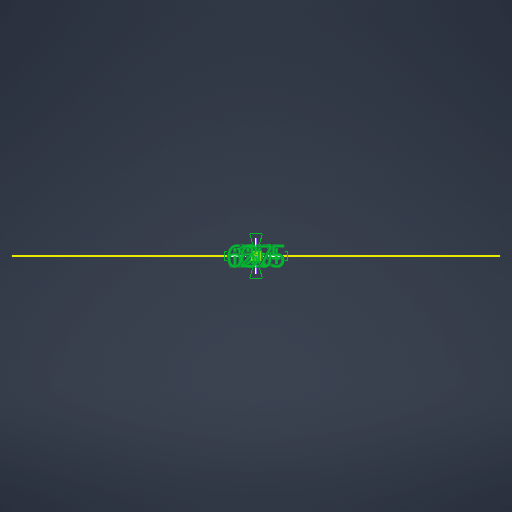
# Autodesk Inventor part: Sensor_Mount
Saved by Autodesk Inventor 2027.1 (Build 311270010, 270A)
## iProperties
Created: 2026-09-08
Part Number: Sensor_Mount
Material: Generic
Document SubType Name: Modeling
Designer: Jacob Parker
Density: 1 g/cm^3
Appearance: Default
Author: Jacob Parker
Autodesk Inventor part; units mm, degrees
ref_plane "YZ Plane" through (0, 0, 0) normal (1, 0, 0) x (0, 1, 0)
ref_plane "XZ Plane" through (0, 0, 0) normal (0, 1, 0) x (-1, 0, 0)
ref_plane "XY Plane" through (0, 0, 0) normal (0, 0, 1) x (1, 0, 0)
sketch "SKbase" plane through (0, 0, 0) normal (0, 1, 0) x (-1, 0, 0)
  line L0 (27.5, 100) -> (-27.5, 100)
  line L1 (-27.5, 100) -> (-27.5, -64)
  line L2 (-27.5, -64) -> (27.5, -64)
  line L3 (27.5, -64) -> (27.5, 100)
  point P0 (0, 0)
  point P1 (27.5, 18)
  dimension "d0" = 55
  dimension "d1" = 164
  constraints: 8 end point, 2 parallel, 1 horizontal, 1 midpoint, 1 other
  measures "d0" distance of L2.end L1.end
  measures "d1" distance of L2.end L0.start
extrude "EXbase" add sketch "SKbase" along normal blind 18
sketch "SKmounting_holes" plane through (0, 0, 0) normal (0, 1, 0) x (1, 0, 0)
  line L0 (0, 288563.516) -> (0, -288614.916) projected
  line L1 (-38.5, -19) -> (38.5, -19)
  line L2 (0, -288601.516) -> (0, 288576.916)
  line L3 (-27.5, 64) -> (-27.5, -100) projected
  line L4 (-27.5, -100) -> (27.5, -100) projected
  point P0 (0, 0)
  point P1 (-12.5, -94)
  point P2 (-12.5, 56)
  point P3 (12.5, -94)
  point P4 (12.5, 56)
  dimension "d10" = 15
  dimension "d11" = 6
  dimension "d113" = 75
  constraints: 3 vertical alignment, 2 end point, 2 symmetric about line, 3 other
  measures "d10" distance from line of L3 point (-12.5, -94)
  measures "d11" distance from line of L4 point (-12.5, -94)
hole "EXmounting_holes" at (-12.5, 0, 94) at (12.5, 0, 94) at (-12.5, 0, -56) at (12.5, 0, -56) direction (0, 1, 0) diameter 7 end through all
sketch "SKLayout" plane through (0, 18, 0) normal (0, 1, 0) x (1, 0, 0)
  line L0 (-27.5, -86.5) -> (27.5, -86.5)
  line L1 (-27.5, -59.5) -> (27.5, -59.5)
  line L2 (-27.5, 0.5) -> (27.5, 0.5)
  line L3 (-27.5, 64) -> (-27.5, -100) projected
  line L4 (-27.5, 64) -> (27.5, 64)
  line L5 (27.5, -100) -> (27.5, 64) projected
  line L6 (-27.5, -100) -> (27.5, -100) projected
  point P0 (27.5, 64)
  dimension "d81" = 27
  dimension "d82" = 60
  dimension "d109" = 63.5
  dimension "d112" = 13.5
  constraints: 8 end point, 2 point on line, 1 horizontal
  measures "d81" distance between parallel lines of L0 L1
  measures "d82" distance between parallel lines of L1 L2
  measures "d109" distance between parallel lines of L2 L4
  measures "d112" distance between parallel lines of L6 L0
sketch "SKbolt_head_hole" plane through (0, 18, 0) normal (0, 1, 0) x (1, 0, 0)
  point P0 (0, 0)
  point P1 (12.5, 56)
  point P2 (-12.5, 56)
  point P3 (-12.5, -94)
  point P4 (12.5, -94)
hole "Hbolt_head_hole" at (-12.5, 18, 94) at (12.5, 18, 94) at (-12.5, 18, -56) at (12.5, 18, -56) direction (0, -1, 0) diameter 11 depth 5
sketch "SKprint_head_holes" plane through (0, 18, 0) normal (0, 1, 0) x (1, 0, 0)
  circle A0 centre (20, -37) radius 3 projected
  circle A1 centre (-20, -53) radius 3 projected
  circle A2 centre (-20, -21) radius 3 projected
  point P0 (0, 0)
hole "Hprint_head_holes" at (-20, 18, 53) at (-20, 18, 21) at (20, 18, 37) direction (0, -1, 0) diameter 6 end through all
sketch "SKnut_place" plane through (0, 0, 0) normal (0, -1, 0) x (1, 0, 0)
  circle A0 centre (20, 37) radius 3 projected
  line L0 (20, 31.5) -> (15.2369, 34.25)
  line L1 (15.2369, 34.25) -> (15.2369, 39.75)
  line L2 (15.2369, 39.75) -> (20, 42.5)
  line L3 (20, 42.5) -> (24.7631, 39.75)
  line L4 (24.7631, 39.75) -> (24.7631, 34.25)
  line L5 (24.7631, 34.25) -> (20, 31.5)
  circle A1 centre (-20, 53) radius 3 projected
  line L6 (-20, 47.5) -> (-24.7631, 50.25)
  line L7 (-24.7631, 50.25) -> (-24.7631, 55.75)
  line L8 (-24.7631, 55.75) -> (-20, 58.5)
  line L9 (-20, 58.5) -> (-15.2369, 55.75)
  line L10 (-15.2369, 55.75) -> (-15.2369, 50.25)
  line L11 (-15.2369, 50.25) -> (-20, 47.5)
  circle A2 centre (-20, 21) radius 3 projected
  line L12 (-20, 15.5) -> (-24.7631, 18.25)
  line L13 (-24.7631, 18.25) -> (-24.7631, 23.75)
  line L14 (-24.7631, 23.75) -> (-20, 26.5)
  line L15 (-20, 26.5) -> (-15.2369, 23.75)
  line L16 (-15.2369, 23.75) -> (-15.2369, 18.25)
  line L17 (-15.2369, 18.25) -> (-20, 15.5)
  point P0 (0, 0)
  point P1 (20, 37)
  point P2 (-20, 53)
  point P3 (-20, 21)
  dimension "d97" = 11
  dimension "d99" = 11
  dimension "d137" = 11
  constraints: 36 end point, 3 coincident, 39 other
  measures "d97" distance of L0.start L2.end
  measures "d99" distance of L8.end L6.start
  measures "d137" distance of L14.end L12.start
extrude "EXnut_place" cut sketch "SKnut_place" against normal blind 5.5 contours A0 | L0 L1 L2 L3 L4 L5 | A1 | L6 L7 L8 L9 L10 L11 | A2 | L12 L13 L14 L15 L16 L17
sketch "Sketch13" plane through (0, 0, 0) normal (0, -1, 0) x (1, 0, 0)
  line L0 (27.5, 100) -> (27.5, -64) projected
  line L1 (7.5, -48.5) -> (-27.5, -48.5) projected
  line L2 (7.5, 1.5) -> (7.5, -48.5) projected
  line L3 (-27.5, 1.5) -> (7.5, 1.5) projected
  line L4 (-27.5, -64) -> (-27.5, 100) projected
  point P0 (-27.5, -46.5)
  point P1 (27.5, -64)
  point P2 (27.5, -64)
extrude "Extrusion8" cut sketch "Sketch13" against normal blind 12
sketch "Sketch16" plane through (0, 12, 0) normal (0, -1, 0) x (1, 0, 0)
  circle A0 centre (0.4313, -3.5) radius 2 projected
  circle A1 centre (0.4313, -43.5) radius 2 projected
  point P0 (0, 0)
hole "Hole6" at (0.4313, 12, -3.5) at (0.4313, 12, -43.5) direction (0, 1, 0) diameter 6 end through all
sketch "Sketch18" plane through (27.5, 0, 100) normal (1, 0, 0) x (0, 0, -1)
  line L0 (63.6887, 16.6372) -> (192.0696, 16.6372) construction
  line L1 (192.0696, 16.6372) -> (192.0696, 29.4271) construction
  line L2 (192.0696, 29.4271) -> (63.6887, 29.4271) construction
  line L3 (63.6887, 29.4271) -> (63.6887, 16.6372) construction
  spline S0 degree 2 poles (67.4143, 14.8794) (67.4143, 14.5501) (67.1797, 13.9573) (66.9697, 13.7514) knots 0 0 0 1 2 2 2
  spline S1 degree 2 poles (66.9697, 13.7514) (66.7062, 13.4921) (65.9941, 13.2245) (65.4507, 13.2245) knots 0 0 0 1 2 2 2
  line L4 (65.4507, 13.2245) -> (64.8784, 13.2245)
  line L5 (64.8784, 13.2245) -> (64.8784, 11.3308)
  line L6 (64.8784, 11.3308) -> (64.2033, 11.3308)
  line L7 (64.2033, 11.3308) -> (64.2033, 16.4108)
  line L8 (64.2033, 16.4108) -> (65.4795, 16.4108)
  spline S2 degree 2 poles (65.4795, 16.4108) (65.9323, 16.4108) (66.5663, 16.2626) (66.8092, 16.0938) knots 0 0 0 1 2 2 2
  spline S3 degree 2 poles (66.8092, 16.0938) (67.0932, 15.9003) (67.4143, 15.3034) (67.4143, 14.8794) knots 0 0 0 1 2 2 2
  spline S4 degree 2 poles (66.7104, 14.8588) (66.7104, 15.1223) (66.5292, 15.5093) (66.344, 15.6328) knots 0 0 0 1 2 2 2
  spline S5 degree 2 poles (66.344, 15.6328) (66.1834, 15.7398) (65.7553, 15.8262) (65.4383, 15.8262) knots 0 0 0 1 2 2 2
  line L9 (65.4383, 15.8262) -> (64.8784, 15.8262)
  line L10 (64.8784, 15.8262) -> (64.8784, 13.8008)
  line L11 (64.8784, 13.8008) -> (65.3395, 13.8008)
  spline S6 degree 2 poles (65.3395, 13.8008) (65.7512, 13.8008) (66.2575, 13.9326) (66.4222, 14.1055) knots 0 0 0 1 2 2 2
  spline S7 degree 2 poles (66.4222, 14.1055) (66.5745, 14.2578) (66.7104, 14.6159) (66.7104, 14.8588) knots 0 0 0 1 2 2 2
  line L12 (68.6617, 11.3308) -> (68.0195, 11.3308)
  line L13 (68.0195, 11.3308) -> (68.0195, 15.1429)
  line L14 (68.0195, 15.1429) -> (68.6617, 15.1429)
  line L15 (68.6617, 15.1429) -> (68.6617, 11.3308)
  line L16 (68.707, 15.7768) -> (67.9783, 15.7768)
  line L17 (67.9783, 15.7768) -> (67.9783, 16.4438)
  line L18 (67.9783, 16.4438) -> (68.707, 16.4438)
  line L19 (68.707, 16.4438) -> (68.707, 15.7768)
  line L20 (72.5972, 11.3308) -> (71.955, 11.3308)
  line L21 (71.955, 11.3308) -> (71.955, 13.5044)
  spline S8 degree 2 poles (71.955, 13.5044) (71.955, 13.7679) (71.9056, 14.2207) (71.8315, 14.3566) knots 0 0 0 1 2 2 2
  spline S9 degree 2 poles (71.8315, 14.3566) (71.7533, 14.5007) (71.4734, 14.6406) (71.2346, 14.6406) knots 0 0 0 1 2 2 2
  spline S10 degree 2 poles (71.2346, 14.6406) (70.9958, 14.6406) (70.4895, 14.3854) (70.2466, 14.1796) knots 0 0 0 1 2 2 2
  line L22 (70.2466, 14.1796) -> (70.2466, 11.3308)
  line L23 (70.2466, 11.3308) -> (69.6044, 11.3308)
  line L24 (69.6044, 11.3308) -> (69.6044, 15.1429)
  line L25 (69.6044, 15.1429) -> (70.2466, 15.1429)
  line L26 (70.2466, 15.1429) -> (70.2466, 14.7189)
  spline S11 degree 2 poles (70.2466, 14.7189) (70.5348, 14.9782) (71.0905, 15.2499) (71.4034, 15.2499) knots 0 0 0 1 2 2 2
  spline S12 degree 2 poles (71.4034, 15.2499) (71.9633, 15.2499) (72.5972, 14.5089) (72.5972, 13.805) knots 0 0 0 1 2 2 2
  line L27 (72.5972, 13.805) -> (72.5972, 11.3308)
  spline S13 degree 2 poles (74.6515, 11.2567) (74.1286, 11.2567) (73.54, 11.8536) (73.54, 12.5) knots 0 0 0 1 2 2 2
  line L28 (73.54, 12.5) -> (73.54, 14.6118)
  line L29 (73.54, 14.6118) -> (73.1077, 14.6118)
  line L30 (73.1077, 14.6118) -> (73.1077, 15.1429)
  line L31 (73.1077, 15.1429) -> (73.54, 15.1429)
  line L32 (73.54, 15.1429) -> (73.54, 16.2379)
  line L33 (73.54, 16.2379) -> (74.1822, 16.2379)
  line L34 (74.1822, 16.2379) -> (74.1822, 15.1429)
  line L35 (74.1822, 15.1429) -> (75.3637, 15.1429)
  line L36 (75.3637, 15.1429) -> (75.3637, 14.6118)
  line L37 (75.3637, 14.6118) -> (74.1822, 14.6118)
  line L38 (74.1822, 14.6118) -> (74.1822, 12.7964)
  spline S14 degree 2 poles (74.1822, 12.7964) (74.1822, 12.5082) (74.2027, 12.1912) (74.2727, 12.0554) knots 0 0 0 1 2 2 2
  spline S15 degree 2 poles (74.2727, 12.0554) (74.3304, 11.936) (74.5897, 11.8166) (74.812, 11.8166) knots 0 0 0 1 2 2 2
  spline S16 degree 2 poles (74.812, 11.8166) (74.9685, 11.8166) (75.2607, 11.9113) (75.3266, 11.9401) knots 0 0 0 1 2 2 2
  line L39 (75.3266, 11.9401) -> (75.3637, 11.9401)
  line L40 (75.3637, 11.9401) -> (75.3637, 11.3638)
  spline S17 degree 2 poles (75.3637, 11.3638) (75.1825, 11.3144) (74.812, 11.2567) (74.6515, 11.2567) knots 0 0 0 1 2 2 2
  spline S18 degree 2 poles (77.9613, 11.7343) (77.8831, 11.6766) (77.6196, 11.4708) (77.4961, 11.409) knots 0 0 0 1 2 2 2
  spline S19 degree 2 poles (77.4961, 11.409) (77.3273, 11.3185) (77.0103, 11.2238) (76.7222, 11.2238) knots 0 0 0 1 2 2 2
  spline S20 degree 2 poles (76.7222, 11.2238) (76.4875, 11.2238) (76.0635, 11.4008) (75.9029, 11.5614) knots 0 0 0 1 2 2 2
  spline S21 degree 2 poles (75.9029, 11.5614) (75.7506, 11.7178) (75.5654, 12.1789) (75.5654, 12.4341) knots 0 0 0 1 2 2 2
  spline S22 degree 2 poles (75.5654, 12.4341) (75.5654, 12.8293) (75.8988, 13.3892) (76.2611, 13.5497) knots 0 0 0 1 2 2 2
  spline S23 degree 2 poles (76.2611, 13.5497) (76.5822, 13.6979) (77.4549, 13.8091) (77.9613, 13.8379) knots 0 0 0 1 2 2 2
  line L41 (77.9613, 13.8379) -> (77.9613, 13.9614)
  spline S24 degree 2 poles (77.9613, 13.9614) (77.9613, 14.1837) (77.8254, 14.4595) (77.7019, 14.5377) knots 0 0 0 1 2 2 2
  spline S25 degree 2 poles (77.7019, 14.5377) (77.5784, 14.6159) (77.2244, 14.6653) (77.035, 14.6653) knots 0 0 0 1 2 2 2
  spline S26 degree 2 poles (77.035, 14.6653) (76.8127, 14.6653) (76.2117, 14.5336) (75.9112, 14.406) knots 0 0 0 1 2 2 2
  line L42 (75.9112, 14.406) -> (75.8741, 14.406)
  line L43 (75.8741, 14.406) -> (75.8741, 15.0605)
  spline S27 degree 2 poles (75.8741, 15.0605) (76.0511, 15.1099) (76.7139, 15.2334) (77.0392, 15.2334) knots 0 0 0 1 2 2 2
  spline S28 degree 2 poles (77.0392, 15.2334) (77.4344, 15.2334) (77.9736, 15.1099) (78.1877, 14.9494) knots 0 0 0 1 2 2 2
  spline S29 degree 2 poles (78.1877, 14.9494) (78.3977, 14.793) (78.6035, 14.2948) (78.6035, 13.9367) knots 0 0 0 1 2 2 2
  line L44 (78.6035, 13.9367) -> (78.6035, 11.3308)
  line L45 (78.6035, 11.3308) -> (77.9613, 11.3308)
  line L46 (77.9613, 11.3308) -> (77.9613, 11.7343)
  line L47 (77.9613, 12.2694) -> (77.9613, 13.3274)
  spline S30 degree 2 poles (77.9613, 13.3274) (77.7308, 13.3068) (77.035, 13.2368) (76.8168, 13.171) knots 0 0 0 1 2 2 2
  spline S31 degree 2 poles (76.8168, 13.171) (76.5616, 13.0928) (76.2282, 12.7675) (76.2282, 12.4794) knots 0 0 0 1 2 2 2
  spline S32 degree 2 poles (76.2282, 12.4794) (76.2282, 12.15) (76.5987, 11.8166) (76.9527, 11.8166) knots 0 0 0 1 2 2 2
  spline S33 degree 2 poles (76.9527, 11.8166) (77.2532, 11.8166) (77.7472, 12.0759) (77.9613, 12.2694) knots 0 0 0 1 2 2 2
  line L48 (80.1596, 11.3308) -> (79.5174, 11.3308)
  line L49 (79.5174, 11.3308) -> (79.5174, 15.1429)
  line L50 (79.5174, 15.1429) -> (80.1596, 15.1429)
  line L51 (80.1596, 15.1429) -> (80.1596, 11.3308)
  line L52 (80.2049, 15.7768) -> (79.4762, 15.7768)
  line L53 (79.4762, 15.7768) -> (79.4762, 16.4438)
  line L54 (79.4762, 16.4438) -> (80.2049, 16.4438)
  line L55 (80.2049, 16.4438) -> (80.2049, 15.7768)
  line L56 (81.7569, 11.3308) -> (81.1147, 11.3308)
  line L57 (81.1147, 11.3308) -> (81.1147, 16.6372)
  line L58 (81.1147, 16.6372) -> (81.7569, 16.6372)
  line L59 (81.7569, 16.6372) -> (81.7569, 11.3308)
  line L60 (87.8743, 15.1429) -> (86.4376, 11.3308)
  line L61 (86.4376, 11.3308) -> (85.8612, 11.3308)
  line L62 (85.8612, 11.3308) -> (84.4368, 15.1429)
  line L63 (84.4368, 15.1429) -> (85.1326, 15.1429)
  line L64 (85.1326, 15.1429) -> (86.1741, 12.2077)
  line L65 (86.1741, 12.2077) -> (87.2074, 15.1429)
  line L66 (87.2074, 15.1429) -> (87.8743, 15.1429)
  spline S34 degree 2 poles (91.427, 13.8708) (91.427, 12.5041) (90.6325, 11.2238) (89.805, 11.2238) knots 0 0 0 1 2 2 2
  spline S35 degree 2 poles (89.805, 11.2238) (88.9652, 11.2238) (88.1789, 12.5288) (88.1789, 13.8667) knots 0 0 0 1 2 2 2
  spline S36 degree 2 poles (88.1789, 13.8667) (88.1789, 15.2417) (88.9734, 16.5137) (89.805, 16.5137) knots 0 0 0 1 2 2 2
  spline S37 degree 2 poles (89.805, 16.5137) (90.6407, 16.5137) (91.427, 15.1964) (91.427, 13.8708) knots 0 0 0 1 2 2 2
  spline S38 degree 2 poles (90.5543, 12.3229) (90.6531, 12.5741) (90.7354, 13.348) (90.7354, 13.8708) knots 0 0 0 1 2 2 2
  spline S39 degree 2 poles (90.7354, 13.8708) (90.7354, 14.3936) (90.6531, 15.1635) (90.5501, 15.4228) knots 0 0 0 1 2 2 2
  spline S40 degree 2 poles (90.5501, 15.4228) (90.4472, 15.6822) (90.0891, 15.9497) (89.805, 15.9497) knots 0 0 0 1 2 2 2
  spline S41 degree 2 poles (89.805, 15.9497) (89.521, 15.9497) (89.1546, 15.6822) (89.0475, 15.4146) knots 0 0 0 1 2 2 2
  spline S42 degree 2 poles (89.0475, 15.4146) (88.9446, 15.1552) (88.8705, 14.3648) (88.8705, 13.8667) knots 0 0 0 1 2 2 2
  spline S43 degree 2 poles (88.8705, 13.8667) (88.8705, 13.3315) (88.9364, 12.6152) (89.0434, 12.3353) knots 0 0 0 1 2 2 2
  spline S44 degree 2 poles (89.0434, 12.3353) (89.1422, 12.0718) (89.5086, 11.7878) (89.805, 11.7878) knots 0 0 0 1 2 2 2
  spline S45 degree 2 poles (89.805, 11.7878) (90.085, 11.7878) (90.4513, 12.0554) (90.5543, 12.3229) knots 0 0 0 1 2 2 2
  line L67 (93.1684, 11.3308) -> (92.3533, 11.3308)
  line L68 (92.3533, 11.3308) -> (92.3533, 12.3024)
  line L69 (92.3533, 12.3024) -> (93.1684, 12.3024)
  line L70 (93.1684, 12.3024) -> (93.1684, 11.3308)
  line L71 (97.071, 11.3308) -> (94.5927, 11.3308)
  line L72 (94.5927, 11.3308) -> (94.5927, 11.8495)
  line L73 (94.5927, 11.8495) -> (95.5149, 11.8495)
  line L74 (95.5149, 11.8495) -> (95.5149, 15.254)
  line L75 (95.5149, 15.254) -> (94.5927, 15.254)
  line L76 (94.5927, 15.254) -> (94.5927, 15.7192)
  spline S46 degree 2 poles (94.5927, 15.7192) (95.1156, 15.7192) (95.6096, 16.0156) (95.6425, 16.4273) knots 0 0 0 1 2 2 2
  line L77 (95.6425, 16.4273) -> (96.1694, 16.4273)
  line L78 (96.1694, 16.4273) -> (96.1694, 11.8495)
  line L79 (96.1694, 11.8495) -> (97.071, 11.8495)
  line L80 (97.071, 11.8495) -> (97.071, 11.3308)
  line L81 (99.0964, 11.3308) -> (98.2813, 11.3308)
  line L82 (98.2813, 11.3308) -> (98.2813, 12.3024)
  line L83 (98.2813, 12.3024) -> (99.0964, 12.3024)
  line L84 (99.0964, 12.3024) -> (99.0964, 11.3308)
  spline S47 degree 2 poles (101.4923, 15.9292) (101.3071, 15.9292) (100.9407, 15.8386) (100.7637, 15.7686) knots 0 0 0 1 2 2 2
  spline S48 degree 2 poles (100.7637, 15.7686) (100.599, 15.6986) (100.3561, 15.5504) (100.2614, 15.4846) knots 0 0 0 1 2 2 2
  line L85 (100.2614, 15.4846) -> (100.2203, 15.4846)
  line L86 (100.2203, 15.4846) -> (100.2203, 16.205)
  spline S49 degree 2 poles (100.2203, 16.205) (100.4426, 16.3244) (101.2041, 16.5179) (101.5458, 16.5179) knots 0 0 0 1 2 2 2
  spline S50 degree 2 poles (101.5458, 16.5179) (101.8916, 16.5179) (102.4062, 16.3779) (102.6162, 16.2297) knots 0 0 0 1 2 2 2
  spline S51 degree 2 poles (102.6162, 16.2297) (102.8385, 16.0691) (103.069, 15.6039) (103.069, 15.2911) knots 0 0 0 1 2 2 2
  spline S52 degree 2 poles (103.069, 15.2911) (103.069, 14.8712) (102.5174, 14.2372) (102.1304, 14.1549) knots 0 0 0 1 2 2 2
  line L87 (102.1304, 14.1549) -> (102.1304, 14.1055)
  spline S53 degree 2 poles (102.1304, 14.1055) (102.291, 14.0725) (102.6573, 13.9243) (102.8138, 13.7761) knots 0 0 0 1 2 2 2
  spline S54 degree 2 poles (102.8138, 13.7761) (102.9702, 13.6321) (103.1678, 13.171) (103.1678, 12.8375) knots 0 0 0 1 2 2 2
  spline S55 degree 2 poles (103.1678, 12.8375) (103.1678, 12.4958) (102.9332, 11.9154) (102.7191, 11.6931) knots 0 0 0 1 2 2 2
  spline S56 degree 2 poles (102.7191, 11.6931) (102.4968, 11.4626) (101.8669, 11.2238) (101.4676, 11.2238) knots 0 0 0 1 2 2 2
  spline S57 degree 2 poles (101.4676, 11.2238) (101.0848, 11.2238) (100.3355, 11.409) (100.0803, 11.5367) knots 0 0 0 1 2 2 2
  line L88 (100.0803, 11.5367) -> (100.0803, 12.2571)
  line L89 (100.0803, 12.2571) -> (100.1297, 12.2571)
  spline S58 degree 2 poles (100.1297, 12.2571) (100.3438, 12.1006) (101.0683, 11.8125) (101.4264, 11.8125) knots 0 0 0 1 2 2 2
  spline S59 degree 2 poles (101.4264, 11.8125) (101.6364, 11.8125) (102.0563, 11.9442) (102.1963, 12.0965) knots 0 0 0 1 2 2 2
  spline S60 degree 2 poles (102.1963, 12.0965) (102.3321, 12.2488) (102.4762, 12.6111) (102.4762, 12.8869) knots 0 0 0 1 2 2 2
  spline S61 degree 2 poles (102.4762, 12.8869) (102.4762, 13.1627) (102.3157, 13.5209) (102.1716, 13.6238) knots 0 0 0 1 2 2 2
  spline S62 degree 2 poles (102.1716, 13.6238) (102.0275, 13.7267) (101.6364, 13.805) (101.4059, 13.805) knots 0 0 0 1 2 2 2
  line L90 (101.4059, 13.805) -> (101.1177, 13.805)
  line L91 (101.1177, 13.805) -> (101.1177, 14.3689)
  line L92 (101.1177, 14.3689) -> (101.3441, 14.3689)
  spline S63 degree 2 poles (101.3441, 14.3689) (101.8011, 14.3689) (102.3774, 14.8053) (102.3774, 15.2211) knots 0 0 0 1 2 2 2
  spline S64 degree 2 poles (102.3774, 15.2211) (102.3774, 15.4146) (102.2292, 15.6904) (102.1098, 15.7727) knots 0 0 0 1 2 2 2
  spline S65 degree 2 poles (102.1098, 15.7727) (101.9822, 15.8592) (101.6693, 15.9292) (101.4923, 15.9292) knots 0 0 0 1 2 2 2
  spline S66 degree 2 poles (63.9192, 6.3959) (63.9192, 6.787) (64.1745, 7.4375) (64.3968, 7.6721) knots 0 0 0 1 2 2 2
  spline S67 degree 2 poles (64.3968, 7.6721) (64.6067, 7.8985) (65.2201, 8.1496) (65.533, 8.1496) knots 0 0 0 1 2 2 2
  spline S68 degree 2 poles (65.533, 8.1496) (65.8829, 8.1496) (66.451, 7.915) (66.661, 7.6927) knots 0 0 0 1 2 2 2
  spline S69 degree 2 poles (66.661, 7.6927) (66.9244, 7.4128) (67.2126, 6.5071) (67.2126, 5.8114) knots 0 0 0 1 2 2 2
  spline S70 degree 2 poles (67.2126, 5.8114) (67.2126, 5.1815) (66.9286, 4.0535) (66.6527, 3.6789) knots 0 0 0 1 2 2 2
  spline S71 degree 2 poles (66.6527, 3.6789) (66.3604, 3.2837) (65.5371, 2.8679) (64.9361, 2.8679) knots 0 0 0 1 2 2 2
  spline S72 degree 2 poles (64.9361, 2.8679) (64.8002, 2.8679) (64.4915, 2.8967) (64.3597, 2.9379) knots 0 0 0 1 2 2 2
  line L93 (64.3597, 2.9379) -> (64.3597, 3.5925)
  line L94 (64.3597, 3.5925) -> (64.3927, 3.5925)
  spline S73 degree 2 poles (64.3927, 3.5925) (64.4791, 3.5431) (64.8414, 3.4566) (65.0266, 3.4566) knots 0 0 0 1 2 2 2
  spline S74 degree 2 poles (65.0266, 3.4566) (65.6935, 3.4566) (66.4551, 4.3376) (66.5086, 5.1527) knots 0 0 0 1 2 2 2
  spline S75 degree 2 poles (66.5086, 5.1527) (66.2369, 4.9674) (65.7429, 4.7987) (65.4507, 4.7987) knots 0 0 0 1 2 2 2
  spline S76 degree 2 poles (65.4507, 4.7987) (65.1707, 4.7987) (64.7055, 4.9222) (64.4709, 5.0992) knots 0 0 0 1 2 2 2
  spline S77 degree 2 poles (64.4709, 5.0992) (64.1992, 5.3091) (63.9192, 5.9472) (63.9192, 6.3959) knots 0 0 0 1 2 2 2
  spline S78 degree 2 poles (66.5251, 5.9637) (66.5251, 6.4783) (66.3357, 7.1287) (66.167, 7.3057) knots 0 0 0 1 2 2 2
  spline S79 degree 2 poles (66.167, 7.3057) (66.0188, 7.4704) (65.71, 7.5939) (65.5289, 7.5939) knots 0 0 0 1 2 2 2
  spline S80 degree 2 poles (65.5289, 7.5939) (65.109, 7.5939) (64.6109, 6.9929) (64.6109, 6.4248) knots 0 0 0 1 2 2 2
  spline S81 degree 2 poles (64.6109, 6.4248) (64.6109, 6.1037) (64.7755, 5.6879) (64.9567, 5.5397) knots 0 0 0 1 2 2 2
  spline S82 degree 2 poles (64.9567, 5.5397) (65.0884, 5.4326) (65.4136, 5.3626) (65.603, 5.3626) knots 0 0 0 1 2 2 2
  spline S83 degree 2 poles (65.603, 5.3626) (65.8212, 5.3626) (66.3234, 5.515) (66.5128, 5.6426) knots 0 0 0 1 2 2 2
  spline S84 degree 2 poles (66.5128, 5.6426) (66.5169, 5.692) (66.5251, 5.8608) (66.5251, 5.9637) knots 0 0 0 1 2 2 2
  line L95 (69.9831, 8.2732) -> (67.9948, 1.8635)
  line L96 (67.9948, 1.8635) -> (67.4184, 1.8635)
  line L97 (67.4184, 1.8635) -> (69.3986, 8.2732)
  line L98 (69.3986, 8.2732) -> (69.9831, 8.2732)
  line L99 (73.6758, 2.9667) -> (70.543, 2.9667)
  line L100 (70.543, 2.9667) -> (70.543, 3.6872)
  spline S85 degree 2 poles (70.543, 3.6872) (70.8806, 4.0041) (71.4816, 4.5928) (71.7698, 4.9098) knots 0 0 0 1 2 2 2
  spline S86 degree 2 poles (71.7698, 4.9098) (72.3502, 5.5479) (72.7743, 6.3136) (72.7743, 6.7212) knots 0 0 0 1 2 2 2
  spline S87 degree 2 poles (72.7743, 6.7212) (72.7743, 6.9352) (72.6425, 7.2563) (72.5231, 7.3592) knots 0 0 0 1 2 2 2
  spline S88 degree 2 poles (72.5231, 7.3592) (72.4038, 7.4622) (72.0909, 7.5651) (71.9015, 7.5651) knots 0 0 0 1 2 2 2
  spline S89 degree 2 poles (71.9015, 7.5651) (71.7204, 7.5651) (71.3499, 7.4745) (71.1811, 7.4045) knots 0 0 0 1 2 2 2
  spline S90 degree 2 poles (71.1811, 7.4045) (71.037, 7.3469) (70.7694, 7.1822) (70.6871, 7.1246) knots 0 0 0 1 2 2 2
  line L101 (70.6871, 7.1246) -> (70.65, 7.1246)
  line L102 (70.65, 7.1246) -> (70.65, 7.8491)
  spline S91 degree 2 poles (70.65, 7.8491) (70.86, 7.952) (71.6133, 8.1538) (71.9509, 8.1538) knots 0 0 0 1 2 2 2
  spline S92 degree 2 poles (71.9509, 8.1538) (72.6631, 8.1538) (73.4659, 7.4004) (73.4659, 6.7582) knots 0 0 0 1 2 2 2
  spline S93 degree 2 poles (73.4659, 6.7582) (73.4659, 6.4577) (73.3259, 5.9555) (73.2024, 5.7414) knots 0 0 0 1 2 2 2
  spline S94 degree 2 poles (73.2024, 5.7414) (73.0789, 5.5191) (72.7207, 5.0827) (72.5231, 4.8728) knots 0 0 0 1 2 2 2
  spline S95 degree 2 poles (72.5231, 4.8728) (72.202, 4.5228) (71.4157, 3.7736) (71.1811, 3.5554) knots 0 0 0 1 2 2 2
  line L103 (71.1811, 3.5554) -> (73.6758, 3.5554)
  line L104 (73.6758, 3.5554) -> (73.6758, 2.9667)
  line L105 (77.2326, 2.9667) -> (74.7544, 2.9667)
  line L106 (74.7544, 2.9667) -> (74.7544, 3.4854)
  line L107 (74.7544, 3.4854) -> (75.6765, 3.4854)
  line L108 (75.6765, 3.4854) -> (75.6765, 6.8899)
  line L109 (75.6765, 6.8899) -> (74.7544, 6.8899)
  line L110 (74.7544, 6.8899) -> (74.7544, 7.3551)
  spline S96 degree 2 poles (74.7544, 7.3551) (75.2772, 7.3551) (75.7712, 7.6515) (75.8041, 8.0632) knots 0 0 0 1 2 2 2
  line L111 (75.8041, 8.0632) -> (76.3311, 8.0632)
  line L112 (76.3311, 8.0632) -> (76.3311, 3.4854)
  line L113 (76.3311, 3.4854) -> (77.2326, 3.4854)
  line L114 (77.2326, 3.4854) -> (77.2326, 2.9667)
  line L115 (80.279, 8.2732) -> (78.2906, 1.8635)
  line L116 (78.2906, 1.8635) -> (77.7143, 1.8635)
  line L117 (77.7143, 1.8635) -> (79.6944, 8.2732)
  line L118 (79.6944, 8.2732) -> (80.279, 8.2732)
  line L119 (83.9717, 2.9667) -> (80.8389, 2.9667)
  line L120 (80.8389, 2.9667) -> (80.8389, 3.6872)
  spline S97 degree 2 poles (80.8389, 3.6872) (81.1764, 4.0041) (81.7775, 4.5928) (82.0656, 4.9098) knots 0 0 0 1 2 2 2
  spline S98 degree 2 poles (82.0656, 4.9098) (82.6461, 5.5479) (83.0701, 6.3136) (83.0701, 6.7212) knots 0 0 0 1 2 2 2
  spline S99 degree 2 poles (83.0701, 6.7212) (83.0701, 6.9352) (82.9384, 7.2563) (82.819, 7.3592) knots 0 0 0 1 2 2 2
  spline S100 degree 2 poles (82.819, 7.3592) (82.6996, 7.4622) (82.3867, 7.5651) (82.1974, 7.5651) knots 0 0 0 1 2 2 2
  spline S101 degree 2 poles (82.1974, 7.5651) (82.0162, 7.5651) (81.6457, 7.4745) (81.4769, 7.4045) knots 0 0 0 1 2 2 2
  spline S102 degree 2 poles (81.4769, 7.4045) (81.3329, 7.3469) (81.0653, 7.1822) (80.9829, 7.1246) knots 0 0 0 1 2 2 2
  line L121 (80.9829, 7.1246) -> (80.9459, 7.1246)
  line L122 (80.9459, 7.1246) -> (80.9459, 7.8491)
  spline S103 degree 2 poles (80.9459, 7.8491) (81.1558, 7.952) (81.9092, 8.1538) (82.2468, 8.1538) knots 0 0 0 1 2 2 2
  spline S104 degree 2 poles (82.2468, 8.1538) (82.959, 8.1538) (83.7617, 7.4004) (83.7617, 6.7582) knots 0 0 0 1 2 2 2
  spline S105 degree 2 poles (83.7617, 6.7582) (83.7617, 6.4577) (83.6217, 5.9555) (83.4982, 5.7414) knots 0 0 0 1 2 2 2
  spline S106 degree 2 poles (83.4982, 5.7414) (83.3747, 5.5191) (83.0166, 5.0827) (82.819, 4.8728) knots 0 0 0 1 2 2 2
  spline S107 degree 2 poles (82.819, 4.8728) (82.4979, 4.5228) (81.7116, 3.7736) (81.4769, 3.5554) knots 0 0 0 1 2 2 2
  line L123 (81.4769, 3.5554) -> (83.9717, 3.5554)
  line L124 (83.9717, 3.5554) -> (83.9717, 2.9667)
  spline S108 degree 2 poles (87.8125, 5.5067) (87.8125, 4.14) (87.018, 2.8597) (86.1906, 2.8597) knots 0 0 0 1 2 2 2
  spline S109 degree 2 poles (86.1906, 2.8597) (85.3508, 2.8597) (84.5645, 4.1647) (84.5645, 5.5026) knots 0 0 0 1 2 2 2
  spline S110 degree 2 poles (84.5645, 5.5026) (84.5645, 6.8776) (85.359, 8.1496) (86.1906, 8.1496) knots 0 0 0 1 2 2 2
  spline S111 degree 2 poles (86.1906, 8.1496) (87.0263, 8.1496) (87.8125, 6.8323) (87.8125, 5.5067) knots 0 0 0 1 2 2 2
  spline S112 degree 2 poles (86.9398, 3.9589) (87.0386, 4.21) (87.1209, 4.9839) (87.1209, 5.5067) knots 0 0 0 1 2 2 2
  spline S113 degree 2 poles (87.1209, 5.5067) (87.1209, 6.0296) (87.0386, 6.7994) (86.9357, 7.0587) knots 0 0 0 1 2 2 2
  spline S114 degree 2 poles (86.9357, 7.0587) (86.8328, 7.3181) (86.4746, 7.5857) (86.1906, 7.5857) knots 0 0 0 1 2 2 2
  spline S115 degree 2 poles (86.1906, 7.5857) (85.9065, 7.5857) (85.5401, 7.3181) (85.4331, 7.0505) knots 0 0 0 1 2 2 2
  spline S116 degree 2 poles (85.4331, 7.0505) (85.3302, 6.7911) (85.2561, 6.0007) (85.2561, 5.5026) knots 0 0 0 1 2 2 2
  spline S117 degree 2 poles (85.2561, 5.5026) (85.2561, 4.9674) (85.3219, 4.2511) (85.429, 3.9712) knots 0 0 0 1 2 2 2
  spline S118 degree 2 poles (85.429, 3.9712) (85.5278, 3.7077) (85.8942, 3.4237) (86.1906, 3.4237) knots 0 0 0 1 2 2 2
  spline S119 degree 2 poles (86.1906, 3.4237) (86.4705, 3.4237) (86.8369, 3.6913) (86.9398, 3.9589) knots 0 0 0 1 2 2 2
  line L125 (91.5958, 2.9667) -> (88.463, 2.9667)
  line L126 (88.463, 2.9667) -> (88.463, 3.6872)
  spline S120 degree 2 poles (88.463, 3.6872) (88.8005, 4.0041) (89.4016, 4.5928) (89.6898, 4.9098) knots 0 0 0 1 2 2 2
  spline S121 degree 2 poles (89.6898, 4.9098) (90.2702, 5.5479) (90.6942, 6.3136) (90.6942, 6.7212) knots 0 0 0 1 2 2 2
  spline S122 degree 2 poles (90.6942, 6.7212) (90.6942, 6.9352) (90.5625, 7.2563) (90.4431, 7.3592) knots 0 0 0 1 2 2 2
  spline S123 degree 2 poles (90.4431, 7.3592) (90.3237, 7.4622) (90.0109, 7.5651) (89.8215, 7.5651) knots 0 0 0 1 2 2 2
  spline S124 degree 2 poles (89.8215, 7.5651) (89.6404, 7.5651) (89.2698, 7.4745) (89.1011, 7.4045) knots 0 0 0 1 2 2 2
  spline S125 degree 2 poles (89.1011, 7.4045) (88.957, 7.3469) (88.6894, 7.1822) (88.6071, 7.1246) knots 0 0 0 1 2 2 2
  line L127 (88.6071, 7.1246) -> (88.57, 7.1246)
  line L128 (88.57, 7.1246) -> (88.57, 7.8491)
  spline S126 degree 2 poles (88.57, 7.8491) (88.78, 7.952) (89.5333, 8.1538) (89.8709, 8.1538) knots 0 0 0 1 2 2 2
  spline S127 degree 2 poles (89.8709, 8.1538) (90.5831, 8.1538) (91.3858, 7.4004) (91.3858, 6.7582) knots 0 0 0 1 2 2 2
  spline S128 degree 2 poles (91.3858, 6.7582) (91.3858, 6.4577) (91.2459, 5.9555) (91.1224, 5.7414) knots 0 0 0 1 2 2 2
  spline S129 degree 2 poles (91.1224, 5.7414) (90.9989, 5.5191) (90.6407, 5.0827) (90.4431, 4.8728) knots 0 0 0 1 2 2 2
  spline S130 degree 2 poles (90.4431, 4.8728) (90.122, 4.5228) (89.3357, 3.7736) (89.1011, 3.5554) knots 0 0 0 1 2 2 2
  line L129 (89.1011, 3.5554) -> (91.5958, 3.5554)
  line L130 (91.5958, 3.5554) -> (91.5958, 2.9667)
  spline S131 degree 2 poles (95.4861, 4.6134) (95.4861, 4.2223) (95.2267, 3.5595) (95.0085, 3.3372) knots 0 0 0 1 2 2 2
  spline S132 degree 2 poles (95.0085, 3.3372) (94.7821, 3.1026) (94.214, 2.8597) (93.8723, 2.8597) knots 0 0 0 1 2 2 2
  spline S133 degree 2 poles (93.8723, 2.8597) (93.5306, 2.8597) (92.9666, 3.0902) (92.7526, 3.3208) knots 0 0 0 1 2 2 2
  spline S134 degree 2 poles (92.7526, 3.3208) (92.4891, 3.5966) (92.1927, 4.5228) (92.1927, 5.198) knots 0 0 0 1 2 2 2
  spline S135 degree 2 poles (92.1927, 5.198) (92.1927, 5.8608) (92.4644, 6.927) (92.7485, 7.3222) knots 0 0 0 1 2 2 2
  spline S136 degree 2 poles (92.7485, 7.3222) (93.0243, 7.7092) (93.897, 8.1414) (94.4692, 8.1414) knots 0 0 0 1 2 2 2
  spline S137 degree 2 poles (94.4692, 8.1414) (94.638, 8.1414) (94.9344, 8.1085) (95.0456, 8.0714) knots 0 0 0 1 2 2 2
  line L131 (95.0456, 8.0714) -> (95.0456, 7.4169)
  line L132 (95.0456, 7.4169) -> (95.0168, 7.4169)
  spline S138 degree 2 poles (95.0168, 7.4169) (94.9221, 7.4663) (94.5763, 7.5527) (94.3787, 7.5527) knots 0 0 0 1 2 2 2
  spline S139 degree 2 poles (94.3787, 7.5527) (93.7447, 7.5527) (92.9666, 6.6965) (92.8925, 5.8567) knots 0 0 0 1 2 2 2
  spline S140 degree 2 poles (92.8925, 5.8567) (93.1354, 6.0254) (93.6459, 6.2107) (93.9505, 6.2107) knots 0 0 0 1 2 2 2
  spline S141 degree 2 poles (93.9505, 6.2107) (94.2469, 6.2107) (94.6915, 6.0913) (94.9344, 5.9102) knots 0 0 0 1 2 2 2
  spline S142 degree 2 poles (94.9344, 5.9102) (95.2144, 5.7002) (95.4861, 5.0498) (95.4861, 4.6134) knots 0 0 0 1 2 2 2
  spline S143 degree 2 poles (94.7945, 4.5846) (94.7945, 4.8975) (94.6298, 5.3215) (94.4486, 5.4697) knots 0 0 0 1 2 2 2
  spline S144 degree 2 poles (94.4486, 5.4697) (94.3128, 5.5767) (93.9752, 5.6467) (93.7982, 5.6467) knots 0 0 0 1 2 2 2
  spline S145 degree 2 poles (93.7982, 5.6467) (93.5594, 5.6467) (93.1107, 5.5026) (92.8925, 5.3668) knots 0 0 0 1 2 2 2
  spline S146 degree 2 poles (92.8925, 5.3668) (92.8884, 5.2927) (92.8802, 5.1527) (92.8802, 5.0457) knots 0 0 0 1 2 2 2
  spline S147 degree 2 poles (92.8802, 5.0457) (92.8802, 4.5187) (93.086, 3.8724) (93.2425, 3.7036) knots 0 0 0 1 2 2 2
  spline S148 degree 2 poles (93.2425, 3.7036) (93.3865, 3.5431) (93.6994, 3.4155) (93.8764, 3.4155) knots 0 0 0 1 2 2 2
  spline S149 degree 2 poles (93.8764, 3.4155) (94.2881, 3.4155) (94.7945, 4) (94.7945, 4.5846) knots 0 0 0 1 2 2 2
  point P0 (100, 0)
  dimension "d9" = 0
  constraints: 2 other
extrude "Extrusion10" cut sketch "Sketch18" against normal blind 5
body "Solid1"
